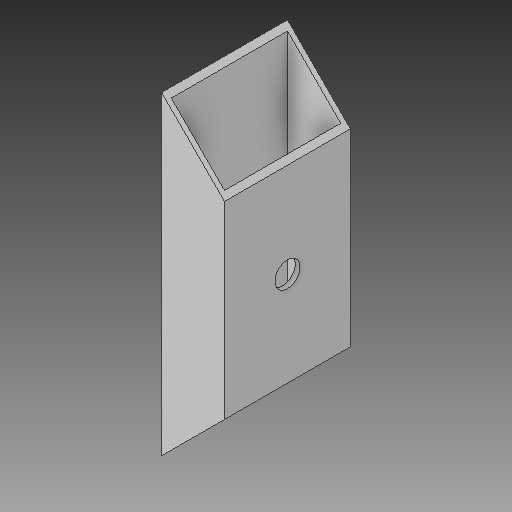
# Autodesk Inventor part: Pipe2
Saved by Autodesk Inventor 2018 (Build 220112000, 112)
## iProperties
Created: 2017-09-09
Part Number: Pipe2
Material: 一般
Document SubType Name: Modeling
Designer: mura5
Density: 1 g/cm^3
Appearance: 既定
Author: mura5
Autodesk Inventor part; units mm, degrees
ref_plane "YZ Plane" through (0, 0, 0) normal (1, 0, 0) x (0, 1, 0)
ref_plane "XZ Plane" through (0, 0, 0) normal (0, 1, 0) x (-1, 0, 0)
ref_plane "XY Plane" through (0, 0, 0) normal (0, 0, 1) x (1, 0, 0)
sketch "スケッチ2" plane through (0, 0, 0) normal (0, 1, 0) x (-1, 0, 0)
  line L0 (15, -30) -> (-15, -30)
  line L1 (-15, -30) -> (-15, 30)
  line L2 (-15, 30) -> (15, 30)
  line L3 (15, 30) -> (15, -30)
  line L4 (15, -30) -> (-15, 30) construction
  line L5 (-15, -30) -> (15, 30) construction
  line L6 (12.7, 27.7) -> (-12.7, 27.7)
  line L7 (-12.7, 27.7) -> (-12.7, -27.7)
  line L8 (-12.7, -27.7) -> (12.7, -27.7)
  line L9 (12.7, -27.7) -> (12.7, 27.7)
  point P0 (0, 0)
  dimension "d7" = 30
  dimension "d8" = 60
  dimension "d9" = 2.3
  constraints: 20 end point, 4 parallel, 2 midpoint, 2 perpendicular, 1 horizontal, 3 other
  measures "d7" distance of L1.end L2.end
  measures "d8" distance of L0.end L1.end
  measures "d9" distance between parallel lines of L2 L6
extrude "押し出し2" add sketch "スケッチ2" along normal mid plane 150
sketch "スケッチ5" plane through (15, -75, -30) normal (1, 0, 0) x (0, 0, -1)
  point P0 (-30, 75)
  point P1 (-30, 75)
  constraints: 1 coincident
hole "穴2" at (15, 0, 0) direction (-1, 0, 0) diameter 12 end through all
chamfer "面取り2" distance 30 angle 45 2 edges at (15, -75, 0) (15, 75, 0)
